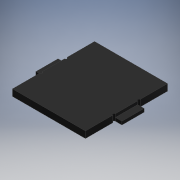
# Autodesk Inventor part: コックピット_2_サブフレーム_4
Saved by Autodesk Inventor 2018 (Build 220112000, 112)
## iProperties
Created: 2016-05-24
Part Number: コックピット_2_サブフレーム_4
Material: アセタール樹脂、黒
Document SubType Name: Modeling
Designer: hiroaki
Density: 1.425 g/cm^3
Appearance: 滑らか - 黒
Mass: 12.6427 g
Surface Area: 58.8321 cm^2
Volume: 8.87208 cm^3
Author: hiroaki
Autodesk Inventor part; units mm, degrees
ref_plane "YZ Plane" through (0, 0, 0) normal (1, 0, 0) x (0, 1, 0)
ref_plane "XZ Plane" through (0, 0, 0) normal (0, 1, 0) x (-1, 0, 0)
ref_plane "XY Plane" through (0, 0, 0) normal (0, 0, 1) x (1, 0, 0)
sketch "スケッチ1" plane through (0, 0, 0) normal (0, 0, 1) x (1, 0, 0)
  line L0 (-28, -31.5) -> (28, -31.5) construction
  line L1 (28, -31.5) -> (28, 31.5) construction
  line L2 (28, 31.5) -> (-28, 31.5) construction
  line L3 (-28, 31.5) -> (-28, -31.5) construction
  line L4 (-28, -31.5) -> (28, 31.5) construction
  line L5 (28, -31.5) -> (-28, 31.5) construction
  line L6 (-28, 10.6) -> (-28, 31.5)
  line L7 (-28, 31.5) -> (28, 31.5)
  line L8 (28, 31.5) -> (28, 10.6)
  line L9 (-28, -10.6) -> (-28, -31.5)
  line L10 (-28, -31.5) -> (28, -31.5)
  line L11 (28, -31.5) -> (28, -10.6)
  line L12 (-28, 8.5) -> (-33, 8.5)
  line L13 (-33, 8.5) -> (-33, -8.5)
  line L14 (-33, -8.5) -> (-28, -8.5)
  line L15 (28, 8.5) -> (33, 8.5)
  line L16 (33, 8.5) -> (33, -8.5)
  line L17 (33, -8.5) -> (28, -8.5)
  line L18 (0, 0) -> (0, 31.5) construction
  line L19 (0, 0) -> (28, 0) construction
  arc A0 (-28, 8.5) -> (-28, 10.6) centre (-28, 9.55) ccw
  arc A1 (-28, -10.6) -> (-28, -8.5) centre (-28, -9.55) ccw
  arc A2 (28, 10.6) -> (28, 8.5) centre (28, 9.55) ccw
  arc A3 (28, -8.5) -> (28, -10.6) centre (28, -9.55) ccw
  dimension "d45" = 63
  dimension "d73" = 56
  dimension "d74" = 1.05
  dimension "d75" = 5
  dimension "d76" = 23
  constraints: 40 end point, 8 perpendicular, 8 point on circle, 4 centre point, 4 midpoint, 4 symmetric about line, 4 tangent, 3 collinear, 3 horizontal, 3 vertical, 3 vertical alignment, 2 parallel, 1 equal radius, 2 other
  measures "d45" distance of L2.end L0.start
  measures "d73" distance of L1.end L2.end
  measures "d74" radius of A0
  measures "d75" distance between parallel lines of L13 L3
  measures "d76" distance between parallel lines of L7 L12
extrude "押し出し1" add sketch "スケッチ1" along normal blind 5
sketch "スケッチ2" plane through (0, 0, 5) normal (0, 0, 1) x (1, 0, 0)
  line L0 (-28, 31.5) -> (-28, 10.6) projected
  line L1 (28, 10.6) -> (28, 31.5) projected
  line L2 (-50.9845, 57.5344) -> (-28, 57.5344)
  line L3 (-28, 57.5344) -> (-28, -57.37)
  line L4 (-28, -57.37) -> (-50.9845, -57.37)
  line L5 (-50.9845, -57.37) -> (-50.9845, 57.5344)
  line L6 (28, 64.7229) -> (65.0267, 64.7229)
  line L7 (65.0267, 64.7229) -> (65.0267, -57.37)
  line L8 (65.0267, -57.37) -> (28, -57.37)
  line L9 (28, -57.37) -> (28, 64.7229)
  point P0 (0, 0)
  constraints: 16 end point, 4 parallel, 2 collinear, 2 horizontal, 2 perpendicular, 1 point on line
extrude "押し出し2" cut sketch "スケッチ2" against normal blind 2.5
equation "\"d45\" = d1"
equation "\"d76\" = d20 + d23"
equation "\"d1\" = 63"
equation "\"d20\" = 8"
equation "\"d23\" = 15"
